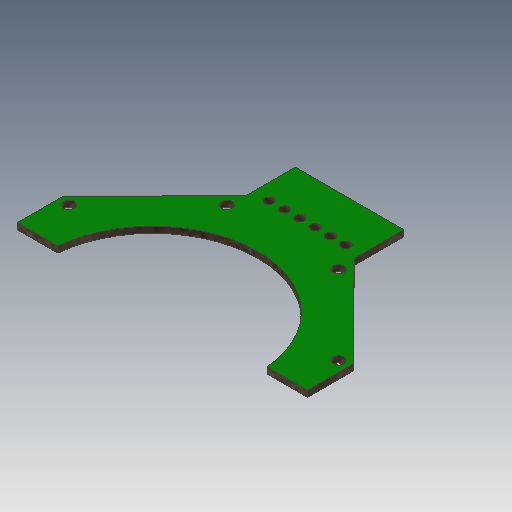
# Autodesk Inventor part: Nema 17 PCB
Saved by Autodesk Inventor 2020.2 (Build 242310000, 310)
## iProperties
Created: 2020-01-21
Part Number: Nema 17 PCB
Material: MDF Medium Density Fiberboard
Document SubType Name: Modeling
Designer: james
Density: 0.8 g/cm^3
Appearance: Cardboard - Corrugated
Mass: 0.228476 g
Surface Area: 8.4661 cm^2
Volume: 0.285596 cm^3
Author: james
Autodesk Inventor part; units mm, degrees
ref_plane "YZ Plane" through (0, 0, 0) normal (1, 0, 0) x (0, 1, 0)
ref_plane "XZ Plane" through (0, 0, 0) normal (0, 1, 0) x (-1, 0, 0)
ref_plane "XY Plane" through (0, 0, 0) normal (0, 0, 1) x (1, 0, 0)
sketch "Sketch11" plane through (0, 0, 0) normal (0, 1, 0) x (-1, 0, 0)
  circle A0 centre (0, 0) radius 13.75
  line L0 (0, -25.75) -> (7.1, -25.75)
  line L1 (7.1, -25.75) -> (7.1, -19.25)
  line L2 (7.1, -19.25) -> (19, -7.25)
  line L3 (19, -7.25) -> (19, -1.25)
  line L4 (19, -1.25) -> (13.6931, -1.25)
  line L5 (0, -25.75) -> (0, -13.75)
  dimension "d82" = 38
  dimension "d83" = 27.5
  dimension "d84" = 14.2
  dimension "d85" = 6
  dimension "d86" = 12
  dimension "d87" = 6.5
  dimension "d88" = 24.5
  constraints: 12 end point, 3 perpendicular, 2 point on circle, 1 centre point, 1 coincident, 1 horizontal, 1 parallel, 1 vertical alignment
  measures "d82" diameter of L3 L5
  measures "d83" diameter of A0
  measures "d84" diameter of L1 L5
  measures "d85" distance of L2.end L3.end
  measures "d86" distance of L0.start L5.end
  measures "d87" distance of L0.end L1.end
  measures "d88" distance between parallel lines of L4 L0
extrude "Extrusion7" add sketch "Sketch11" along normal blind 0.8 contours A0 L4 L3 L2 L1 L0 L5
mirror "Mirror5" about plane through (0, 0, -13.75) normal (1, 0, 0) of "Extrusion7"
sketch "Sketch12" plane through (0, 0.8, 0) normal (0, 1, 0) x (1, 0, 0)
  line L0 (-7.1, 25.75) -> (7.1, 25.75) projected
  line L1 (0, 0) -> (0, 27.3302) construction
  point P0 (-1, 20.25)
  dimension "d91" = 5.5
  dimension "d92" = 1
  constraints: 2 end point, 1 vertical
  measures "d91" distance from line of L0 point (-1, 20.25)
  measures "d92" distance from line of L1 point (-1, 20.25)
hole "Hole5" at (-1, 0.8, -20.25) direction (0, -1, 0) diameter 1.2 end through all
pattern_linear "Rectangular Pattern1" count 6 spacing 2 along (1, 0, 0) of "Hole5" first direction both ways yes
sketch "Sketch13" plane through (0, 0, 0) normal (0, -1, 0) x (1, 0, 0)
  circle A0 centre (-17.65, -6.6609) radius 0.75 projected
  circle A1 centre (-7.3109, -17) radius 0.75 projected
  circle A2 centre (7.3109, -17) radius 0.75 projected
  circle A3 centre (17.65, -6.6609) radius 0.75 projected
  point P0 (0, 0)
extrude "Extrusion8" cut sketch "Sketch13" against normal through all
body "Solid6"
